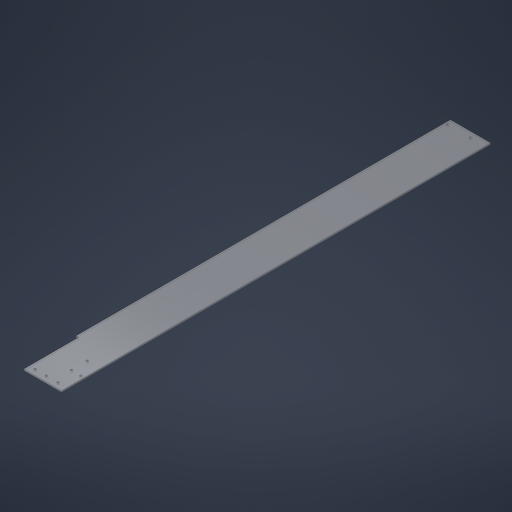
# Autodesk Inventor part: EL2-041
Saved by Autodesk Inventor 2023.4 (Build 274418000, 418)
## iProperties
Created: 2025-03-01
Part Number: EL2-041
Material: Polycarbonate, Clear
Document SubType Name: Sheet Metal
Designer: brand
Density: 1.2 g/cm^3
Sheet Metal Rule: Default
Appearance: Polycarbonate - Clear
Author: brand
Autodesk Inventor part; units mm, degrees
ref_plane "YZ Plane" through (0, 0, 0) normal (1, 0, 0) x (0, 1, 0)
ref_plane "XZ Plane" through (0, 0, 0) normal (0, 1, 0) x (-1, 0, 0)
ref_plane "XY Plane" through (0, 0, 0) normal (0, 0, 1) x (1, 0, 0)
sketch "Sketch1" plane through (0, 0, 0) normal (0, 1, 0) x (-1, 0, 0)
  line L0 (0, -1000.125) -> (-88.9, -1000.125) construction
  line L1 (0, -962.025) -> (-88.9, -962.025) construction
  line L2 (-12.7, 0) -> (-139.7, 0) construction
  line L3 (-6.985, -30.9562) -> (-95.885, -30.9563)
  line L4 (-95.885, -30.9563) -> (-95.885, -983.4562)
  line L5 (-95.885, -983.4562) -> (-6.985, -983.4562)
  line L6 (-6.985, -983.4562) -> (-6.985, -30.9562)
  circle A0 centre (-12.7, -971.55) radius 2.159 construction
  circle A1 centre (-63.5, -971.55) radius 2.159 construction
  circle A2 centre (-3.175, -968.375) radius 1.27 construction
  circle A3 centre (-88.9, -80.9625) radius 2.5527 construction
  circle A4 centre (-12.7, -971.55) radius 5.334 construction
  circle A5 centre (-63.5, -971.55) radius 5.334 construction
  circle A6 centre (-88.9, -80.9625) radius 5.7277 construction
  line L7 (-25.4, -42.8625) -> (-25.4, -971.55) construction
  circle A7 centre (-41.783, -82.804) radius 6.604 construction
  circle A8 centre (-70.866, -82.804) radius 6.604 construction
  circle A9 centre (-70.866, -128.3547) radius 6.604 construction
  line L8 (-41.783, -76.2) -> (-70.866, -76.2) construction
  line L9 (-77.47, -82.804) -> (-77.47, -128.3547) construction
  line L10 (-65.2998, -131.9086) -> (-36.2168, -86.3579) construction
  point P0 (0, 0)
  point P1 (-25.4, -7.9375)
  point P2 (-50.8, -7.9375)
  point P3 (-50.8, -42.8625)
  point P4 (-76.2, -7.9375)
  point P5 (-76.2, -42.8625)
  point P6 (-25.4, -507.2062)
  point P7 (-95.885, -507.2062)
  point P8 (-67.31, -116.6812)
  point P9 (-67.31, -81.7562)
  dimension "d1" = 38.1
  dimension "d2" = 88.9
  dimension "d3" = 1000.125
  dimension "d4" = 12.7
  dimension "d5" = 127
  dimension "d6" = 12.7
  dimension "d7" = 25.4
  dimension "d8" = 25.4
  dimension "d9" = 34.925
  dimension "d10" = 7.9375
  dimension "d11" = 80.9625
  dimension "d12" = 76.2
  dimension "d13" = 6.35
  dimension "d14" = 3.175
  dimension "d15" = 12.7
  dimension "d16" = 63.5
  dimension "d17" = 9.525
  dimension "d18" = 952.5
  dimension "d19" = 4.318
  dimension "d20" = 4.318
  dimension "d21" = 2.54
  dimension "d23" = 5.1054
  dimension "OFF" = 3.175
  dimension "d26" = 3.175
  dimension "d27" = 3.175
  dimension "d28" = 88.9
  dimension "d29" = 6.985
  dimension "d39" = 34.925
  dimension "d40" = 13.208
  dimension "d41" = 13.208
  dimension "d42" = 13.208
  dimension "d43" = 45.5507
  dimension "d44" = 29.083
  dimension "d45" = 82.804
  dimension "d46" = 29.083
  dimension "d47" = 60.325
  dimension "d48" = 50.8
  constraints: 22 end point, 10 centre point, 9 horizontal alignment, 8 vertical alignment, 6 point on circle, 6 tangent, 4 coincident, 3 horizontal, 3 parallel, 2 midpoint, 2 perpendicular
  measures "d1" distance between parallel lines of L0 L1
  measures "d2" distance of L0.start L0.end
  measures "d3" distance between parallel lines of L0 L2
  measures "d4" horizontal distance of L0.start L2.start
  measures "d5" distance of L2.start L2.end
  measures "d6" horizontal distance of L2.start point (-25.4, -7.937)
  measures "d7" distance of point (-25.4, -7.937) point (-50.8, -7.937)
  measures "d8" distance of point (-76.2, -7.937) point (-50.8, -7.937)
  measures "d9" distance of point (-25.4, -7.937) L7.start
  measures "d10" distance from line of L2 point (-25.4, -7.937)
  measures "d11" distance from line of L2 point (-88.9, -80.962)
  measures "d12" horizontal distance of L2.start point (-88.9, -80.962)
  measures "d13" distance from line of L1 point (-3.175, -968.375)
  measures "d14" horizontal distance of L1.start point (-3.175, -968.375)
  measures "d15" horizontal distance of L1.start point (-12.7, -971.55)
  measures "d16" horizontal distance of L1.start point (-63.5, -971.55)
  measures "d17" distance from line of L1 point (-63.5, -971.55)
  measures "d18" distance of L5.end L3.start
  measures "d19" diameter of A0
  measures "d20" diameter of A1
  measures "d21" diameter of A2
  measures "d23" diameter of A3
  measures "OFF" radial gap between concentric circles of A0 A4
  measures "d26" radial gap between concentric circles of A1 A5
  measures "d27" radial gap between concentric circles of A3 A6
  measures "d28" distance of L4.end L5.end
  measures "d29" distance from line of point (0, 0) L6
  measures "d39" distance of point (-67.31, -81.756) point (-67.31, -116.681)
  measures "d40" diameter of A7
  measures "d41" diameter of A8
  measures "d42" diameter of A9
  measures "d43" distance of A8.centre A9.centre
  measures "d44" distance of A7.centre A8.centre
  measures "d45" vertical distance of A7.centre L2.start
  measures "d46" horizontal distance of L2.start A7.centre
  measures "d47" distance from line of L6 point (-67.31, -81.756)
  measures "d48" distance from line of L3 point (-67.31, -81.756)
extrude "Plate1" add sketch "Sketch1" against normal blind 3.175
hole "Hole1" at (25.4, 0, -42.8625) at (25.4, 0, -7.9375) at (50.8, 0, -7.9375) at (50.8, 0, -42.8625) at (76.2, 0, -7.9375) at (76.2, 0, -42.8625) at (88.9, 0, -80.9625) at (12.7, 0, -971.55) at (63.5, 0, -971.55) at (3.175, 0, -968.375) direction (0, -1, 0) diameter 5.1054 end through all clearance for "Flat Head Machine Screw (82)" size "#10" standard "Ansi Unified Screw Threads"
hole "Hole2" at (67.31, 0, -116.6812) at (67.31, 0, -81.7562) direction (0, -1, 0) diameter 5.1054 end through all clearance for "Flat Head Machine Screw (82)" size "#10" standard "Ansi Unified Screw Threads"
sketch "Sketch2" plane through (0, 0, 0) normal (0, 1, 0) x (1, 0, 0)
  circle A0 centre (67.31, 116.6812) radius 2.5527 construction
  circle A1 centre (67.31, 81.7562) radius 2.5527 construction
  circle A2 centre (63.5, 971.55) radius 2.5527 construction
  circle A3 centre (88.9, 80.9625) radius 2.5527 construction
  circle A4 centre (25.4, 42.8625) radius 2.5527 construction
  circle A5 centre (50.8, 42.8625) radius 2.5527 construction
  circle A6 centre (76.2, 42.8625) radius 2.5527 construction
  circle A7 centre (12.7, 971.55) radius 2.5527 construction
  line L0 (95.885, 983.4562) -> (95.885, 30.9563) construction
  line L1 (95.885, 30.9563) -> (6.985, 30.9562) construction
  line L2 (6.985, 30.9562) -> (6.985, 983.4562) construction
  line L3 (6.985, 983.4562) -> (95.885, 983.4562) construction
  line L4 (0, 152.4) -> (12.7, 152.4)
  line L5 (12.7, 152.4) -> (12.7, 0)
  line L6 (12.7, 0) -> (0, 0)
  line L7 (0, 0) -> (0, 152.4)
  dimension "d56" = 152.4
  dimension "d58" = 12.7
  constraints: 8 end point, 2 parallel, 1 coincident, 1 horizontal, 1 perpendicular
  measures "d56" distance of L4.end L5.end
  measures "d58" distance of L4.start L4.end
extrude "Extrusion1" cut sketch "Sketch2" against normal through all
equation "\"d8\" = d7"
equation "\"d20\" = d19"
equation "\"d26\" = OFF"
equation "\"d27\" = OFF"
equation "\"d41\" = d40"
equation "\"d42\" = d40"
equation "\"d37\" = Thickness"
equation "\"d31\" = Thickness"
equation "\"BendRadius\" = Thickness"
equation "\"BendReliefWidth\" = Thickness"
equation "\"BendReliefDepth\" = 0.5 * Thickness"
equation "\"CornerReliefSize\" = 4 * Thickness"
equation "\"MinimumRemnant\" = 2 * Thickness"
equation "\"TransitionRadius\" = BendRadius"
equation "\"JacobiRadiusSize\" = BendRadius"
equation "\"GapSize\" = Thickness"
equation "\"Thickness\" = 3.175"
body "Solid1"
